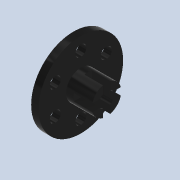
# Autodesk Inventor part: CircleArm
Saved by Autodesk Inventor 2021.2 (Build 252289000, 289)
## iProperties
Created: 2020-12-25
Part Number: CircleArm
Material: Generic
Document SubType Name: Modeling
Designer: Hagihara Yuya
Density: 1 g/cm^3
Appearance: 滑らか - 黒
Author: Hagihara Yuya
Autodesk Inventor part; units mm, degrees
ref_plane "YZ Plane" through (0, 0, 0) normal (1, 0, 0) x (0, 1, 0)
ref_plane "XZ Plane" through (0, 0, 0) normal (0, 1, 0) x (-1, 0, 0)
ref_plane "XY Plane" through (0, 0, 0) normal (0, 0, 1) x (1, 0, 0)
sketch "スケッチ1" plane through (0, 0, 0) normal (1, 0, 0) x (0, 1, 0)
  circle A0 centre (0, 0) radius 11.5
  dimension "d0" = 23
  constraints: 1 centre point, 1 coincident
  measures "d0" diameter of A0
extrude "押し出し1" add sketch "スケッチ1" along normal blind 2
sketch "スケッチ4" plane through (0, 0, 0) normal (-1, 0, 0) x (0, 0, 1)
  circle A0 centre (0, 0) radius 4
  dimension "d22" = 8
  constraints: 1 centre point, 1 coincident
  measures "d22" diameter of A0
extrude "押し出し2" add sketch "スケッチ4" along normal blind 7
sketch "スケッチ5" plane through (-7, 0, 0) normal (-1, 0, 0) x (0, 0, 1)
  line L0 (-4, 1) -> (4, 1)
  line L1 (4, 1) -> (4, -1)
  line L2 (4, -1) -> (-4, -1)
  line L3 (-4, -1) -> (-4, 1)
  line L4 (-1, 4) -> (1, 4)
  line L5 (1, 4) -> (1, -4)
  line L6 (1, -4) -> (-1, -4)
  line L7 (-1, -4) -> (-1, 4)
  circle A0 centre (0, 0) radius 4 projected
  circle A1 centre (0, 0) radius 2
  point P0 (0, 4)
  point P1 (4, 0)
  point P2 (1, 0)
  point P3 (0, 1)
  point P4 (1, 1)
  point P5 (-1, 1)
  point P6 (-1, -1)
  point P7 (1, -1)
  point P8 (-1, 1.7321)
  point P9 (-1.7321, 1)
  point P10 (1.7321, 1)
  point P11 (1, 1.7321)
  point P12 (-1.7321, -1)
  point P13 (-1, -1.7321)
  point P14 (1, -1.7321)
  point P15 (1.7321, -1)
  dimension "d25" = 2
  dimension "d26" = 2
  dimension "d29" = 4
  constraints: 16 end point, 4 midpoint, 4 parallel, 2 horizontal, 2 horizontal alignment, 2 perpendicular, 2 tangent, 2 vertical alignment, 1 centre point, 1 coincident
  measures "d25" distance of L0.end L1.end
  measures "d26" distance of L5.end L6.end
  measures "d29" diameter of A1
extrude "押し出し3" cut sketch "スケッチ5" against normal blind 5 contours L0 A0 L3 | L0 A1 L2 A0 | A0 L2 L3 | A1 L7 L0 | L0 L7 L2 A1 | A0 L5 A1 L7 | L7 L4 A0 | L7 A1 L5 L0 | L0 L5 L2 L7 | L2 L7 A1 | L4 L5 A0 | A0 L6 L7 | L7 A1 L5 A0 | L5 A1 L0 | L0 A1 L2 L5 | L2 L5 A1 L7 | A0 L5 L6 | L0 A0 L2 A1 | L2 A1 L5 | L0 L1 A0 | L1 L2 A0
sketch "スケッチ2" plane through (2, 0, 0) normal (1, 0, 0) x (0, 0, -1)
  point P0 (0, 0)
  point P1 (0, 0)
  constraints: 1 coincident
hole "穴1" at (2, 0, 0) direction (-1, 0, 0) diameter 3 end through all
sketch "スケッチ3" plane through (2, 0, 0) normal (1, 0, 0) x (0, 0, -1)
  point P0 (0, 0)
  point P1 (8, 0)
  point P2 (4, 6.9282)
  point P3 (-4, 6.9282)
  point P4 (-8, 0)
  point P5 (-4, -6.9282)
  point P6 (4, -6.9282)
  dimension "d12" = 360
  dimension "d14" = 16
  constraints: 1 horizontal alignment, 7 other
  measures "d14" distance of point (8, 0) point (-8, 0)
hole "穴2" at (2, 0, -8) at (2, 6.9282, -4) at (2, 6.9282, 4) at (2, 0, 8) at (2, -6.9282, 4) at (2, -6.9282, -4) direction (-1, 0, 0) diameter 3 end through all
equation "\"d25\" = d26"
